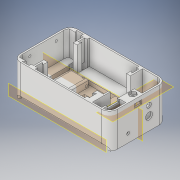
# Autodesk Inventor part: Base
Saved by Autodesk Inventor 2019.3 (Build 233278000, 278)
## iProperties
Created: 2019-01-26
Part Number: Base
Material: PC/ABS Plastic
Document SubType Name: Modeling
Designer: Jared
Density: 0.357273 g/cm^3
Appearance: Smooth - White
Author: Jared
Autodesk Inventor part; units mm, degrees
ref_plane "YZ Plane" through (0, 0, 0) normal (1, 0, 0) x (0, 1, 0)
ref_plane "XZ Plane" through (0, 0, 0) normal (0, 1, 0) x (-1, 0, 0)
ref_plane "XY Plane" through (0, 0, 0) normal (0, 0, 1) x (1, 0, 0)
sketch "Sketch1" plane through (0, 0, 0) normal (0, 1, 0) x (-1, 0, 0)
  line L0 (0, 0) -> (125, 0)
  line L1 (125, 0) -> (125, -74)
  line L2 (125, -74) -> (0, -74)
  line L3 (0, -74) -> (0, 0)
  dimension "d0" = 125
  dimension "d1" = 74
  constraints: 8 end point, 2 parallel, 1 horizontal, 1 perpendicular
  measures "d0" distance of L1.end L2.end
  measures "d1" distance of L0.end L1.end
extrude "Extrusion1" add sketch "Sketch1" along normal blind 3
sketch "Sketch2" plane through (0, 3, 0) normal (0, 1, 0) x (1, 0, 0)
  line L0 (-125, 0) -> (0, 0) projected
  line L1 (0, 0) -> (0, 74) projected
  line L2 (0, 74) -> (-125, 74) projected
  line L3 (-125, 74) -> (-125, 0) projected
  line L4 (-125, 74) -> (-125, 0) projected
  line L5 (-75, 42.5) -> (-50, 42.5)
  line L6 (-50, 42.5) -> (-50, 31.5)
  line L7 (-50, 31.5) -> (-75, 31.5)
  line L8 (-75, 31.5) -> (-75, 42.5)
  line L9 (0, 0) -> (0, 74) projected
  dimension "d8" = 11
  dimension "d9" = 25
  dimension "d10" = 31.5
  dimension "d110" = 50
  constraints: 8 end point, 2 parallel, 1 horizontal, 1 perpendicular
  measures "d8" distance of L5.end L6.end
  measures "d9" distance of L5.start L5.end
  measures "d10" distance between parallel lines of L0 L7
  measures "d110" distance between parallel lines of L1 L6
extrude "Extrusion2" cut sketch "Sketch2" against normal up to next contours L5 L6 L7 L8
sketch "Sketch5" plane through (0, 3, 0) normal (0, 1, 0) x (1, 0, 0)
  line L0 (-75, 31.5) -> (-75, 42.5) projected
  line L1 (-50, 42.5) -> (-50, 31.5) projected
  line L2 (-80, 21.5) -> (-102, 21.5)
  line L3 (-80, 52.5) -> (-102, 52.5)
  line L4 (-50, 31.5) -> (-75, 31.5) projected
  line L5 (-75, 42.5) -> (-50, 42.5) projected
  line L6 (-80, 52.5) -> (-80, 37)
  line L7 (-80, 37) -> (-80, 21.5)
  line L8 (-102, 52.5) -> (-102, 21.5)
  line L9 (-45, 52.5) -> (-31.3245, 52.5)
  line L10 (-30, 21.5) -> (-45, 21.5)
  line L11 (-45, 21.5) -> (-45, 52.5)
  line L12 (-23, 27.9226) -> (-23, 47.9226)
  line L13 (-23, 27.9226) -> (-30, 21.5)
  line L14 (-23, 47.9226) -> (-31.3245, 52.5)
  point P0 (0, 0)
  dimension "d101" = 10
  dimension "d102" = 5
  dimension "d103" = 22
  dimension "d238" = 31
  dimension "d239" = 15
  dimension "d240" = 10
  dimension "d241" = 5
  dimension "d249" = 31
  dimension "d250" = 22
  dimension "d251" = 20
  constraints: 22 end point, 3 equal length, 3 vertical, 1 collinear, 1 horizontal, 1 parallel, 1 perpendicular
  measures "d101" distance between parallel lines of L3 L5
  measures "d102" distance between parallel lines of L0 L6
  measures "d103" distance of L3.start L3.end
  measures "d238" distance of L3.end L2.end
  measures "d239" distance of L10.start L10.end
  measures "d240" distance between parallel lines of L9 L5
  measures "d241" distance between parallel lines of L11 L1
  measures "d249" distance between parallel lines of L9 L10
  measures "d250" distance between parallel lines of L11 L12
  measures "d251" distance of L12.start L12.end
extrude "Extrusion6" add sketch "Sketch5" along normal blind 10 contours L2 L8 L3 L6 L7 | L9 L14 L12 L13 L10 L11
sketch "Sketch3" plane through (0, 0, 0) normal (0, 1, 0) x (1, 0, 0)
  line L0 (-50, 31.5) -> (-50, 42.5) projected
  circle A0 centre (-32, 37) radius 8
  line L1 (-50, 42.5) -> (-50, 31.5) projected
  line L2 (-50, 37) -> (-32, 37)
  line L3 (-75, 31.5) -> (-75, 42.5) projected
  line L4 (-75, 42.5) -> (-50, 42.5) projected
  line L5 (-50, 42.5) -> (-50, 31.5) projected
  line L6 (-50, 31.5) -> (-75, 31.5) projected
  line L7 (-125, 0) -> (0, 0) projected
  line L8 (0, 0) -> (0, 74) projected
  line L9 (0, 74) -> (-125, 74) projected
  line L10 (-125, 74) -> (-125, 0) projected
  line L11 (-75, 42.5) -> (-75, 31.5) projected
  line L12 (-75, 37) -> (-93, 37)
  circle A1 centre (-93, 37) radius 8
  dimension "d27" = 16
  dimension "d29" = 18
  dimension "d243" = 18
  dimension "d244" = 16
  constraints: 4 end point, 2 centre point, 2 horizontal, 2 midpoint, 1 coincident
  measures "d27" diameter of A0
  measures "d29" distance of L2.start L2.end
  measures "d243" distance of L12.start L12.end
  measures "d244" diameter of A1
extrude "Extrusion4" cut sketch "Sketch3" along normal blind 7 contours A0 | A1
ref_plane "Work Plane2" through (-125, 0, 0) normal (0, 0, 1) x (1, 0, 0)
sketch "Sketch13" plane through (-125, 0, 0) normal (0, 0, 1) x (1, 0, 0)
  line L0 (125, 0) -> (0, 0) projected
  line L1 (114.5, 0) -> (10.5, 0)
  line L2 (114.5, 0) -> (114.5, -4.75)
  arc A0 (119.25, -4.75) -> (114.5, 0) centre (114.5, -4.75) ccw
  line L3 (10.5, 0) -> (10.5, -4.75)
  arc A1 (10.5, 0) -> (5.75, -4.75) centre (10.5, -4.75) ccw
  line L4 (114.5, -4.75) -> (119.25, -4.75)
  line L5 (10.5, -4.75) -> (5.75, -4.75)
  line L6 (119.25, -4.75) -> (125, -4.75)
  line L7 (125, 0) -> (125, 3) projected
  line L8 (125, 0) -> (125, -4.75)
  line L9 (5.75, -4.75) -> (0, -4.75)
  line L10 (0, 0) -> (0, -4.75)
  point P0 (125, 8)
  dimension "d104" = 4.75
  dimension "d105" = 4.75
  dimension "d106" = 104
  dimension "d107" = 10.5
  constraints: 18 end point, 4 horizontal, 4 point on circle, 3 vertical, 2 centre point, 2 coincident, 2 point on line, 1 perpendicular
  measures "d104" distance of L1.start L2.end
  measures "d105" distance of L1.end L3.end
  measures "d106" distance of L1.start L1.end
  measures "d107" distance of L0.start L1.start
extrude "Extrusion10" add sketch "Sketch13" against normal up to surface (74 mm away) contours L8 L6 A0 L0 | A1 L9 L10 L0
fillet "Fillet2" radius 10 4 edges at (0, -0.875, -74) (0, -0.875, 0) (-125, -0.875, -74) (-125, -0.875, 0)
sketch "Sketch18" plane through (0, 3, 0) normal (0, 1, 0) x (1, 0, 0)
  line L0 (-115, 2) -> (-10, 2)
  line L1 (-123, 10) -> (-123, 64)
  line L2 (-115, 72) -> (-10, 72)
  line L3 (0, 10) -> (0, 64) projected
  arc A0 (0, 64) -> (-10, 74) centre (-10, 64) ccw projected
  line L4 (-10, 74) -> (-115, 74) projected
  line L5 (-125, 64) -> (-125, 10) projected
  arc A1 (-115, 74) -> (-125, 64) centre (-115, 64) ccw projected
  arc A2 (-125, 10) -> (-115, 0) centre (-115, 10) ccw projected
  line L6 (-115, 0) -> (-10, 0) projected
  line L7 (-2, 64) -> (-2, 10)
  arc A3 (-2, 64) -> (-10, 72) centre (-10, 64) ccw
  arc A4 (-115, 72) -> (-123, 64) centre (-115, 64) ccw
  arc A5 (-123, 10) -> (-115, 2) centre (-115, 10) ccw
  arc A6 (-10, 2) -> (-2, 10) centre (-10, 10) ccw
  arc A7 (-10, 0) -> (0, 10) centre (-10, 10) ccw projected
  point P0 (0, 0)
  point P1 (-2, 2)
  point P2 (-121, 2)
  point P3 (-2, 70)
  dimension "d159" = 8
  dimension "d160" = 2
  dimension "d161" = 2
  dimension "d162" = 2
  dimension "d163" = 2
  constraints: 10 point on circle, 8 end point, 8 tangent, 4 centre point, 3 equal radius, 2 point on line, 2 vertical, 1 horizontal, 1 perpendicular
  measures "d159" radius of A3
  measures "d160" distance between parallel lines of L4 L2
  measures "d161" distance between parallel lines of L3 L7
  measures "d162" distance between parallel lines of L5 L1
  measures "d163" distance between parallel lines of L6 L0
extrude "Extrusion14" add sketch "Sketch18" along normal blind 37
sketch "Sketch21" plane through (0, 3, 0) normal (0, 1, 0) x (1, 0, 0)
  line L0 (-115, 2) -> (-10, 2) projected
  line L1 (-10, 2) -> (-10, 25)
  line L2 (-26, 2) -> (-26, 25)
  line L3 (-26, 25) -> (-10, 25)
  line L4 (-10, 25) -> (-2, 25)
  line L5 (-2, 10) -> (-2, 64) projected
  arc A0 (-10, 2) -> (-2, 10) centre (-10, 10) ccw projected
  point P0 (0, 0)
  dimension "d168" = 23
  dimension "d169" = 16
  constraints: 8 end point, 2 horizontal, 2 point on line, 1 vertical
  measures "d168" distance between parallel lines of L0 L3
  measures "d169" distance between parallel lines of L2 L1
extrude "Extrusion16" add sketch "Sketch21" along normal blind 3
sketch "Sketch22" plane through (0, 6, 0) normal (0, 1, 0) x (1, 0, 0)
  line L0 (-10, 2) -> (-26, 2) projected
  line L1 (-2, 25) -> (-26, 25) projected
  line L2 (-26, 25) -> (-26, 2) projected
  line L3 (-10, 2) -> (-26, 2) projected
  line L4 (-24, 2) -> (-24, 25)
  line L5 (-12, 25) -> (-12, 2)
  arc A0 (-10, 2) -> (-2, 10) centre (-10, 10) ccw projected
  line L6 (-2, 25) -> (-2, 10) projected
  line L7 (-26, 25) -> (-2, 25) projected
  line L8 (-10, 23) -> (-10, 2)
  line L9 (-10, 23) -> (-2, 23)
  line L10 (-2, 25) -> (-2, 10) projected
  point P0 (0, 0)
  dimension "d173" = 2
  dimension "d280" = 12
  dimension "d281" = 2
  constraints: 8 end point, 5 point on line, 3 perpendicular, 1 vertical
  measures "d173" distance between parallel lines of L2 L4
  measures "d280" distance between parallel lines of L4 L5
  measures "d281" distance between parallel lines of L7 L9
extrude "Extrusion17" add sketch "Sketch22" along normal up to surface (34 mm away) contours L0 L5 L1 L6 L9 L8 | L0 L2 L1 L4
ref_plane "Work Plane4" through (-75, 3, -37) normal (0, 0, 1) x (1, 0, 0)
sketch "Sketch25" plane through (-80, 3, -52.5) normal (-1, 0, 0) x (0, 0, 1)
  circle A0 centre (2.5, 3) radius 1.5
  line L0 (0, 0) -> (31, 0) projected
  line L1 (0, 0) -> (0, 10) projected
  line L2 (31, 10) -> (0, 10) projected
  line L3 (31, 0) -> (31, 10) projected
  point P0 (52.5, -3)
  dimension "d189" = 3
  dimension "d247" = 2.5
  dimension "d248" = 3
  constraints: 1 centre point
  measures "d189" diameter of A0
  measures "d247" distance from line of A0.centre L1
  measures "d248" distance from line of L0 A0.centre
extrude "Extrusion19" cut sketch "Sketch25" along normal blind 4 contours A0
sketch "Sketch23" plane through (0, 6, 0) normal (0, 1, 0) x (1, 0, 0)
  line L0 (-24, 25) -> (-24, 2) projected
  line L1 (-12, 2) -> (-24, 2) projected
  line L2 (-24, 2) -> (-24, 25) projected
  line L3 (-24, 19) -> (-12, 19)
  line L4 (-12, 2) -> (-12, 25) projected
  line L5 (-24, 24) -> (-12, 24)
  line L6 (-12, 25) -> (-24, 25) projected
  line L7 (-12, 2) -> (-12, 25) projected
  point P0 (0, 0)
  point P1 (-12, 22.125)
  point P2 (-24.25, 22.125)
  dimension "d179" = 17
  dimension "d180" = 5
  constraints: 4 end point, 2 point on line, 1 horizontal, 1 perpendicular, 3 other
  measures "d179" distance between parallel lines of L1 L3
  measures "d180" distance between parallel lines of L3 L5
extrude "Extrusion18" cut sketch "Sketch23" against normal blind 5 contours L5 L4 L3 L0
fillet "Fillet4" radius 2 10 edges at (-10.2497, -0.0066, -74) (-6.7645, -1.8159, -73.4621) (-114.7503, -0.0066, -74) (-118.2355, -1.8159, -73.4621) (-62.5, 0, -74) (-114.7503, -0.0066, 0) (-118.2355, -1.8159, -0.5379) (-10.2497, -0.0066, 0) (-6.7645, -1.8159, -0.5379) (-62.5, 0, 0)
mirror "Mirror4" about plane through (-75, 3, -37) normal (0, 0, 1) of "Extrusion19"
sketch "Sketch27" plane through (0, 3, 0) normal (0, 1, 0) x (1, 0, 0)
  line L0 (-80, 21.5) -> (-102, 21.5) projected
  line L1 (-102, 52.5) -> (-80, 52.5) projected
  line L2 (-80, 52.5) -> (-80, 21.5) projected
  line L3 (-75, 31.5) -> (-75, 42.5) projected
  line L4 (-75, 42.5) -> (-50, 42.5) projected
  line L5 (-50, 42.5) -> (-50, 31.5) projected
  line L6 (-50, 31.5) -> (-75, 31.5) projected
  line L7 (-26, 2) -> (-26, 25) projected
  line L8 (-26, 25) -> (-2, 25) projected
  line L9 (-2, 25) -> (-2, 64) projected
  arc A0 (-2, 64) -> (-10, 72) centre (-10, 64) ccw projected
  line L10 (-10, 72) -> (-115, 72) projected
  arc A1 (-115, 72) -> (-123, 64) centre (-115, 64) ccw projected
  line L11 (-123, 64) -> (-123, 10) projected
  arc A2 (-123, 10) -> (-115, 2) centre (-115, 10) ccw projected
  line L12 (-115, 2) -> (-26, 2) projected
  line L13 (-106, 5) -> (-113, 5)
  line L14 (-115, 2) -> (-26, 2) projected
  line L15 (-114.5, 2) -> (-10.5, 2) projected
  line L16 (-106, 5) -> (-103, 5)
  arc A3 (-123, 10) -> (-115, 2) centre (-115, 10) ccw projected
  line L17 (-113, 5) -> (-121.245, 5)
  line L18 (-103, 69) -> (-106, 69)
  line L19 (-106, 69) -> (-113, 69)
  arc A4 (-115, 72) -> (-123, 64) centre (-115, 64) ccw projected
  line L20 (-113, 69) -> (-115, 72)
  line L21 (-106, 69) -> (-106, 72)
  line L22 (-113, 69) -> (-121.245, 69)
  line L23 (-115, 72) -> (-10, 72) projected
  line L24 (-103, 72) -> (-103, 56)
  line L25 (-103, 2) -> (-103, 18)
  line L26 (-103, 56) -> (-98, 56)
  line L27 (-103, 18) -> (-98, 18)
  line L28 (-98, 2) -> (-98, 5)
  line L29 (-98, 5) -> (-101, 5)
  line L30 (-98, 18) -> (-98, 12)
  arc A5 (-123, 10) -> (-115, 2) centre (-115, 10) ccw projected
  line L31 (-115, 2) -> (-113, 5)
  line L32 (-106, 5) -> (-106, 2)
  line L33 (-101, 5) -> (-101, 14)
  line L34 (-101, 14) -> (-98, 12)
  line L35 (-98, 56) -> (-98, 62)
  line L36 (-10.5, 72) -> (-114.5, 72) projected
  line L37 (-98, 72) -> (-98, 69)
  line L38 (-98, 69) -> (-101, 69)
  line L39 (-101, 69) -> (-101, 60)
  line L40 (-101, 60) -> (-98, 62)
  line L41 (-34, 56) -> (-34, 62)
  line L42 (-34, 62) -> (-31, 60)
  line L43 (-34, 56) -> (-29, 56)
  line L44 (-29, 56) -> (-29, 72)
  line L45 (-10, 72) -> (-115, 72) projected
  line L46 (-31, 60) -> (-31, 69)
  line L47 (-31, 69) -> (-34, 69)
  line L48 (-34, 69) -> (-34, 72)
  line L49 (-34, 18) -> (-26, 18)
  line L50 (-34, 18) -> (-34, 12)
  line L51 (-34, 12) -> (-31, 14)
  line L52 (-31, 14) -> (-31, 5)
  line L53 (-31, 5) -> (-34, 5)
  line L54 (-34, 5) -> (-34, 2)
  line L55 (-102, 21.5) -> (-102, 52.5) projected
  line L56 (-30, 21.5) -> (-45, 21.5) projected
  line L57 (-45, 21.5) -> (-45, 52.5) projected
  line L58 (-45, 52.5) -> (-31.3245, 52.5) projected
  line L59 (-23, 27.9226) -> (-30, 21.5) projected
  line L60 (-31.3245, 52.5) -> (-23, 47.9226) projected
  line L61 (-23, 47.9226) -> (-23, 27.9226) projected
  point P0 (0, 0)
  point P1 (-103, 2)
  dimension "d193" = 3
  dimension "d195" = 7
  dimension "d199" = 3
  dimension "d200" = 7
  dimension "d201" = 3
  dimension "d204" = 16
  dimension "d205" = 16
  dimension "d206" = 5
  dimension "d207" = 5
  dimension "d208" = 3
  dimension "d209" = 3
  dimension "d210" = 6
  dimension "d212" = 9
  dimension "d213" = 5
  dimension "d214" = 3
  dimension "d215" = 20
  dimension "d216" = 20
  dimension "d217" = 6
  dimension "d218" = 3
  dimension "d219" = 3
  dimension "d220" = 9
  dimension "d221" = 5
  dimension "d222" = 6
  dimension "d223" = 64
  dimension "d224" = 5
  dimension "d225" = 3
  dimension "d226" = 3
  dimension "d227" = 5
  dimension "d228" = 16
  dimension "d229" = 9
  dimension "d232" = 3
  dimension "d233" = 3
  dimension "d234" = 16
  dimension "d235" = 6
  dimension "d236" = 9
  dimension "d237" = 64
  constraints: 74 end point, 14 point on line, 13 perpendicular, 8 vertical, 6 horizontal, 2 parallel, 2 point on circle, 3 other
  measures "d193" distance between parallel lines of L12 L13
  measures "d195" distance of L13.start L13.end
  measures "d199" distance of L18.start L18.end
  measures "d200" distance of L18.end L19.end
  measures "d201" distance between parallel lines of L10 L18
  measures "d204" distance of L24.start L24.end
  measures "d205" distance of L25.start L25.end
  measures "d206" distance of L24.end L26.end
  measures "d207" distance of L25.end L27.end
  measures "d208" distance of L28.start L28.end
  measures "d209" distance of L28.end L29.end
  measures "d210" distance of L27.end L30.end
  measures "d212" distance of L29.end L33.end
  measures "d213" distance between parallel lines of L25 L28
  measures "d214" distance of L13.start L16.end
  measures "d215" distance between parallel lines of L25 L11
  measures "d216" distance between parallel lines of L11 L24
  measures "d217" distance of L26.end L35.end
  measures "d218" distance of L37.start L37.end
  measures "d219" distance of L37.end L38.end
  measures "d220" distance of L38.end L39.end
  measures "d221" distance between parallel lines of L24 L37
  measures "d222" distance of L41.start L41.end
  measures "d223" distance between parallel lines of L35 L41
  measures "d224" distance of L41.start L43.end
  measures "d225" distance between parallel lines of L41 L46
  measures "d226" distance of L47.end L48.end
  measures "d227" distance between parallel lines of L44 L48
  measures "d228" distance between parallel lines of L36 L43
  measures "d229" distance of L42.end L46.end
  measures "d232" distance between parallel lines of L54 L52
  measures "d233" distance of L53.end L54.end
  measures "d234" distance between parallel lines of L12 L49
  measures "d235" distance of L49.start L50.end
  measures "d236" distance of L51.end L52.end
  measures "d237" distance between parallel lines of L30 L50
extrude "Extrusion20" add sketch "Sketch27" along normal up to surface (37 mm away) contours L12 L54 L53 L52 L51 L50 L49 L7 | L12 L25 L27 L30 L34 L33 L29 L28 | L12 L32 L16 L25 | A2 L17 L31 | L44 L43 L41 L42 L46 L47 L48 L10 | L37 L38 L39 L40 L35 L26 L24 L10 | L24 L18 L21 L10 | A1 L20 L22
chamfer "Chamfer2" distance 6 angle 45 1 edges at (-23, 13, -37.9226)
fillet "Fillet5" radius 2 10 edges at (-37.5, 13, -21.5) (-38.1622, 13, -52.5) (-26, 10, -25.1701) (-26, 10, -49.5722) (-91, 13, -21.5) (-80, 13, -37) (-91, 13, -52.5) (-102, 13, -37) (-45, 13, -37) (-23, 7, -37.9226)
sketch "Sketch28" plane through (0, -4.75, -10) normal (1, 0, 0) x (0, 0, -1)
  line L0 (0, 0) -> (0, 44.75) projected
  line L1 (0, 0) -> (54, 0) projected
  line L2 (54, 44.75) -> (54, 0) projected
  line L3 (0, 44.75) -> (54, 44.75) projected
  line L4 (62, 7.75) -> (62, 44.75) projected
  circle A0 centre (41, 16.75) radius 4.5
  circle A1 centre (41, 28.75) radius 3.125
  point P0 (-10, 4.75)
  dimension "d257" = 21
  dimension "d258" = 16.75
  dimension "d259" = 9
  dimension "d306" = 12
  dimension "d307" = 6.25
  dimension "d308" = 21
  constraints: 2 centre point, 1 coincident
  measures "d257" distance from line of point (41, 16.75) L4
  measures "d258" distance from line of L1 point (41, 16.75)
  measures "d259" diameter of A0
  measures "d306" distance of A1.centre A0.centre
  measures "d307" diameter of A1
  measures "d308" distance from line of L4 A1.centre
extrude "Extrusion21" cut sketch "Sketch28" against normal up to surface (2 mm away) contours A0 | A1
sketch "Sketch29" plane through (-45, 3, -52.5) normal (-1, 0, 0) x (0, 0, 1)
  line L0 (0, 8) -> (31, 8) projected
  line L1 (0, 0) -> (0, 8) projected
  line L2 (31, 0) -> (0, 0) projected
  line L3 (31, 0) -> (31, 8) projected
  point P0 (52.5, -3)
  point P1 (28.5, 3)
  dimension "d262" = 2.5
  dimension "d263" = 3
  measures "d262" distance from line of L3 point (28.5, 3)
  measures "d263" distance from line of L2 point (28.5, 3)
hole "Hole3" at (-45, 6, -24) direction (1, 0, 0) diameter 3.75 depth 45 tip angle 118
sketch "Sketch30" plane through (-45, 3, -52.5) normal (-1, 0, 0) x (0, 0, 1)
  circle A0 centre (28.5, 3) radius 1.875 projected
  line L0 (0, 8) -> (31, 8) projected
  line L1 (0, 0) -> (0, 8) projected
  line L2 (31, 0) -> (0, 0) projected
  line L3 (31, 0) -> (31, 8) projected
  point P0 (52.5, -3)
  point P1 (2.5, 3)
  dimension "d271" = 2.5
  dimension "d272" = 3
  measures "d271" distance from line of L1 point (2.5, 3)
  measures "d272" distance from line of L2 point (2.5, 3)
hole "Hole4" at (-45, 6, -50) direction (1, 0, 0) diameter 3.75 depth 43
sketch "Sketch31" plane through (0, 40, 0) normal (0, 1, 0) x (1, 0, 0)
  line L0 (-12, 25) -> (-12, 2) projected
  line L1 (-10, 2) -> (-10, 23) projected
  line L2 (-2, 25) -> (-12, 25) projected
  line L3 (-10, 7) -> (-12, 7)
  line L4 (-10, 22) -> (-12, 22)
  point P0 (0, 0)
  dimension "d282" = 15
  dimension "d283" = 5
  constraints: 4 end point, 4 point on line, 2 perpendicular
  measures "d282" distance between parallel lines of L4 L3
  measures "d283" distance from line of L1.start L3
extrude "Extrusion22" cut sketch "Sketch31" against normal blind 3
sketch "Sketch32" plane through (-103, 3, -18) normal (-1, 0, 0) x (0, 0, 1)
  line L0 (13, 0) -> (13, 37) projected
  line L1 (0, 0) -> (0, 37) projected
  line L2 (13, 0) -> (0, 0) projected
  line L3 (-51, 0) -> (-51, 37) projected
  line L4 (-38, 0) -> (-51, 0) projected
  line L5 (-38, 0) -> (-38, 37) projected
  line L6 (4, 0) -> (4, 10)
  line L7 (4, 10) -> (13, 10)
  line L8 (13, 0) -> (13, 37) projected
  line L9 (-38, 0) -> (-51, 0) projected
  line L10 (-42, 0) -> (-42, 10)
  line L11 (-42, 10) -> (-51, 10)
  line L12 (-51, 0) -> (-51, 37) projected
  line L13 (-51, 37) -> (-38, 37) projected
  line L14 (0, 37) -> (13, 37) projected
  point P0 (18, -3)
  dimension "d286" = 9
  dimension "d287" = 10
  dimension "d288" = 10
  dimension "d289" = 9
  constraints: 8 end point, 4 point on line, 2 perpendicular, 2 vertical
  measures "d286" distance between parallel lines of L6 L0
  measures "d287" distance of L6.start L6.end
  measures "d288" distance of L10.start L10.end
  measures "d289" distance between parallel lines of L3 L10
extrude "Extrusion23" cut sketch "Sketch32" against normal up to surface (2 mm away) contours L2 L6 L7 L0 | L3 L11 L10 L4
sketch "Sketch33" plane through (0, 3, 0) normal (0, 1, 0) x (1, 0, 0)
  line L0 (-106, 72) -> (-115, 72) projected
  line L1 (-106, 69) -> (-106, 72) projected
  line L2 (-98, 69) -> (-106, 69) projected
  line L3 (-103, 60) -> (-101, 60) projected
  line L4 (-103, 56) -> (-103, 60) projected
  line L5 (-115, 72) -> (-113, 69) projected
  line L6 (-113, 69) -> (-121.245, 69) projected
  line L7 (-123, 64) -> (-123, 10) projected
  arc A0 (-121.245, 69) -> (-123, 64) centre (-115, 64) ccw projected
  arc A1 (-123, 10) -> (-121.245, 5) centre (-115, 10) ccw projected
  line L8 (-106, 2) -> (-115, 2) projected
  line L9 (-113, 5) -> (-115, 2) projected
  line L10 (-121.245, 5) -> (-113, 5) projected
  line L11 (-106, 5) -> (-98, 5) projected
  line L12 (-106, 2) -> (-106, 5) projected
  line L13 (-98, 12) -> (-101, 14) projected
  line L14 (-103, 14) -> (-101, 14) projected
  line L15 (-103, 14) -> (-103, 18) projected
  line L16 (-101, 60) -> (-98, 62) projected
  line L17 (-107, 60) -> (-113, 60)
  line L18 (-113, 60) -> (-113, 69)
  line L19 (-103, 14) -> (-113, 14)
  line L20 (-113, 5) -> (-121.245, 5) projected
  line L21 (-113, 14) -> (-113, 5)
  line L22 (-98, 62) -> (-98, 56) projected
  line L23 (-98, 72) -> (-98, 69) projected
  line L24 (-34, 72) -> (-98, 72) projected
  line L25 (-98, 18) -> (-98, 12) projected
  line L26 (-98, 2) -> (-34, 2) projected
  line L27 (-98, 5) -> (-98, 2) projected
  line L28 (-34, 2) -> (-34, 5) projected
  line L29 (-34, 12) -> (-34, 18) projected
  line L30 (-34, 56) -> (-34, 62) projected
  line L31 (-34, 69) -> (-34, 72) projected
  line L32 (-34, 62) -> (-31, 60) projected
  line L33 (-34, 56) -> (-98, 56)
  line L34 (-80, 52.5) -> (-102, 52.5) projected
  line L35 (-98, 18) -> (-34, 18)
  line L36 (-34, 5) -> (-31, 5) projected
  line L37 (-98, 5) -> (-98, 12)
  line L38 (-98, 62) -> (-98, 69)
  line L39 (-112, 60) -> (-112, 14)
  line L40 (-107, 60) -> (-107, 14)
  line L41 (-102, 52.5) -> (-112, 52.5)
  line L42 (-31, 69) -> (-34, 69) projected
  line L43 (-31, 60) -> (-31, 69) projected
  line L44 (-31, 5) -> (-31, 14) projected
  line L45 (-31, 14) -> (-34, 12) projected
  line L46 (-102, 21.5) -> (-102, 52.5) projected
  line L47 (-103, 18) -> (-103, 5) projected
  line L48 (-102, 21.5) -> (-103, 18)
  line L49 (-103, 14) -> (-103, 18)
  line L50 (-102, 21.5) -> (-102, 52.5)
  point P0 (0, 0)
  point P1 (-107, 52.5)
  dimension "d294" = 14
  dimension "d295" = 5
  dimension "d298" = 7.5
  dimension "d299" = 9
  constraints: 28 end point, 6 point on line, 5 perpendicular, 3 horizontal, 2 collinear, 2 vertical, 1 midpoint, 1 parallel
  measures "d294" distance between parallel lines of L39 L38
  measures "d295" distance between parallel lines of L40 L39
  measures "d298" distance between parallel lines of L41 L17
  measures "d299" distance of L17.end L5.end
extrude "Extrusion26" add sketch "Sketch33" along normal blind 5 contours L18 L17 L39 L19 L21 L10 A1 L7 A0 L6 | L41 L46 L48 L15 L19 L40 | L25 L35 L29 L45 L44 L36 L28 L26 L27 L37 | L38 L23 L24 L31 L42 L43 L32 L30 L33 L22
sketch "Sketch34" plane through (0, 3, 0) normal (0, 1, 0) x (1, 0, 0)
  line L0 (-2, 25) -> (-2, 64) projected
  line L1 (-31.3245, 52.5) -> (-23, 47.9226) projected
  line L2 (-10, 72) -> (-29, 72) projected
  arc A0 (-2, 64) -> (-10, 72) centre (-10, 64) ccw projected
  line L3 (-29, 72) -> (-29, 56) projected
  line L4 (-23.5858, 38.75) -> (-2, 38.75)
  line L5 (-23.5858, 36.75) -> (-2, 36.75)
  line L6 (-23, 47.9226) -> (-23, 27.9226) projected
  line L7 (-23.5858, 46.7399) -> (-23.5858, 28.8018) projected
  line L8 (-23.5858, 38.75) -> (-23.5858, 36.75)
  point P0 (0, 0)
  point P1 (-23, 38.75)
  point P2 (-23, 36.75)
  dimension "d302" = 33.25
  dimension "d303" = 2
  constraints: 6 end point, 6 point on line, 1 horizontal, 1 perpendicular, 1 vertical
  measures "d302" distance between parallel lines of L2 L4
  measures "d303" distance between parallel lines of L5 L4
extrude "Extrusion27" add sketch "Sketch34" along normal up to surface (4.5858 mm away)
sketch "Sketch35" plane through (0, 13, 0) normal (0, 1, 0) x (1, 0, 0)
  line L0 (-100, 50.5) -> (-82, 50.5)
  line L1 (-43, 50.5) -> (-29.1715, 50.5)
  line L2 (-29.026, 23.5) -> (-43, 23.5)
  line L3 (-45, 52.5) -> (-45, 21.5) projected
  line L4 (-80, 52.5) -> (-102, 52.5) projected
  line L5 (-31.3245, 52.5) -> (-45, 52.5) projected
  line L6 (-45, 21.5) -> (-30, 21.5) projected
  line L7 (-29, 49.717) -> (-29, 23.8342) projected
  point P0 (0, 0)
  point P1 (-32, 50.5)
  point P2 (-84.5, 50.5)
  dimension "d318" = 13
  dimension "d319" = 2.5
  dimension "d354" = 2
  dimension "d355" = 2
  dimension "d356" = 2
  dimension "d357" = 14
  constraints: 6 end point, 2 point on line
  measures "d318" distance from line of point (-32, 50.5) L3
  measures "d319" distance of L0.end point (-84.5, 50.5)
  measures "d354" distance between parallel lines of L0 L4
  measures "d355" distance between parallel lines of L1 L5
  measures "d356" distance between parallel lines of L6 L2
  measures "d357" distance from line of L7 L2.end
hole "Hole5" at (-43, 13, -23.5) at (-32, 13, -50.5) at (-84.5, 13, -50.5) direction (0, -1, 0) diameter 2.4 depth 6
sketch "Sketch36" plane through (-125, -4.75, -64) normal (-1, 0, 0) x (0, 0, 1)
  line L0 (54, 44.75) -> (54, 0) projected
  line L1 (0, 44.75) -> (54, 44.75) projected
  line L2 (0, 0) -> (0, 44.75) projected
  line L3 (54, 0) -> (0, 0) projected
  circle A0 centre (10, 37.75) radius 1.5
  circle A1 centre (44, 37.75) radius 1.5
  line L4 (10, 37.75) -> (10, 44.75)
  line L5 (44, 37.75) -> (44, 44.75)
  point P0 (64, 4.75)
  dimension "d320" = 3
  dimension "d321" = 7
  dimension "d322" = 10
  dimension "d323" = 10
  constraints: 4 end point, 2 centre point, 2 point on line, 1 equal radius, 1 parallel, 1 perpendicular, 1 vertical
  measures "d320" diameter of A0
  measures "d321" distance of L4.start L4.end
  measures "d322" distance between parallel lines of L2 L4
  measures "d323" distance between parallel lines of L0 L5
extrude "Extrusion28" cut sketch "Sketch36" against normal up to surface (2 mm away) contours A0 | A1
ref_plane "Work Plane5" through (0, 35, 0) normal (0, 1, 0) x (1, 0, 0)
sketch "Sketch37" plane through (0, 35, 0) normal (0, 1, 0) x (1, 0, 0)
  line L0 (-2, 25) -> (-12, 25) projected
  line L1 (-2, 64) -> (-2, 25) projected
  line L2 (-12, 2) -> (-24, 2) projected
  line L3 (-12, 7) -> (-12, 2) projected
  line L4 (-12, 7) -> (-12, 22) projected
  line L5 (-12, 25) -> (-12, 22) projected
  line L6 (-12, 44) -> (-2, 44)
  line L7 (-12, 25) -> (-12, 44)
  line L8 (-29, 72) -> (-10, 72) projected
  circle A0 centre (-7, 37) radius 2
  line L9 (-12, 25) -> (-2, 25)
  line L10 (-2, 44) -> (-2, 25)
  point P0 (0, 0)
  dimension "d328" = 10
  dimension "d330" = 28
  dimension "d339" = 5
  dimension "d340" = 4
  dimension "d342" = 7
  constraints: 8 end point, 2 point on line, 1 centre point, 1 coincident, 1 collinear, 1 perpendicular, 1 vertical
  measures "d328" distance between parallel lines of L1 L7
  measures "d330" distance between parallel lines of L8 L6
  measures "d339" distance from line of L7 point (-7, 37)
  measures "d340" diameter of A0
  measures "d342" distance from line of L6 A0.centre
extrude "Extrusion29" add sketch "Sketch37" along normal blind 2
sketch "Sketch38" plane through (0, 37, 0) normal (0, 1, 0) x (1, 0, 0)
  line L0 (-2, 44) -> (-12, 44) projected
  line L1 (-12, 44) -> (-12, 25) projected
  line L2 (-2, 44) -> (-2, 25) projected
  circle A0 centre (-7, 37) radius 2 projected
  circle A1 centre (-7, 37) radius 2 projected
  line L3 (-11, 39.3094) -> (-7, 41.6188)
  line L4 (-7, 41.6188) -> (-3, 39.3094)
  line L5 (-3, 39.3094) -> (-3, 34.6906)
  line L6 (-3, 34.6906) -> (-7, 32.3812)
  line L7 (-7, 32.3812) -> (-11, 34.6906)
  line L8 (-11, 34.6906) -> (-11, 39.3094)
  line L9 (-2, 25) -> (-12, 25) projected
  point P0 (0, 0)
  point P1 (-7, 37)
  dimension "d341" = 4
  constraints: 12 end point, 1 coincident, 13 other
  measures "d341" distance from line of L8 A0.centre
extrude "Extrusion30" add sketch "Sketch38" along normal blind 3 contours L2 L9 L1 L0
ref_plane "Work Plane7" through (-2, 7.5861, -37) normal (0, 0, -1) x (-1, 0, 0)
ref_plane "Work Plane6" through (-2, 7.5861, -30) normal (0, 0, -1) x (-1, 0, 0)
sketch "Sketch40" plane through (-2, 7.5861, -30) normal (0, 0, -1) x (-1, 0, 0)
  line L0 (0, 0) -> (0, 27.4139) projected
  line L1 (10, 27.4139) -> (0, 27.4139) projected
  line L2 (0, 22.4139) -> (10, 27.4139)
  point P0 (-2, -7.5861)
  dimension "d345" = 5
  constraints: 2 end point, 1 point on line
  measures "d345" vertical distance of L1.start L2.start
extrude "Extrusion31" add sketch "Sketch40" along normal blind 2
mirror "Mirror5" about plane through (-2, 7.5861, -37) normal (0, 0, -1) of "Extrusion31"
sketch "Sketch41" plane through (0, -4.75, -10) normal (1, 0, 0) x (0, 0, -1)
  circle A0 centre (14, 10.75) radius 1.875 projected
  circle A1 centre (41, 28.75) radius 3.125 projected
  circle A2 centre (41, 16.75) radius 4.5 projected
  line L0 (0, 0) -> (0, 44.75) projected
  line L1 (0, 0) -> (54, 0) projected
  line L2 (54, 44.75) -> (54, 0) projected
  line L3 (0, 44.75) -> (54, 44.75) projected
  line L4 (22.5, 39.75) -> (31.5, 39.75)
  line L5 (31.5, 39.75) -> (31.5, 34.75)
  line L6 (31.5, 34.75) -> (22.5, 34.75)
  line L7 (22.5, 34.75) -> (22.5, 39.75)
  point P0 (-10, 4.75)
  dimension "d348" = 9
  dimension "d349" = 5
  dimension "d350" = 5
  dimension "d351" = 22.5
  constraints: 8 end point, 2 parallel, 1 horizontal, 1 perpendicular
  measures "d348" distance of L5.end L6.end
  measures "d349" distance of L4.end L5.end
  measures "d350" distance between parallel lines of L3 L4
  measures "d351" distance between parallel lines of L2 L5
extrude "Extrusion32" cut sketch "Sketch41" against normal up to surface (2 mm away) contours L4 L5 L6 L7
body "Solid1"
